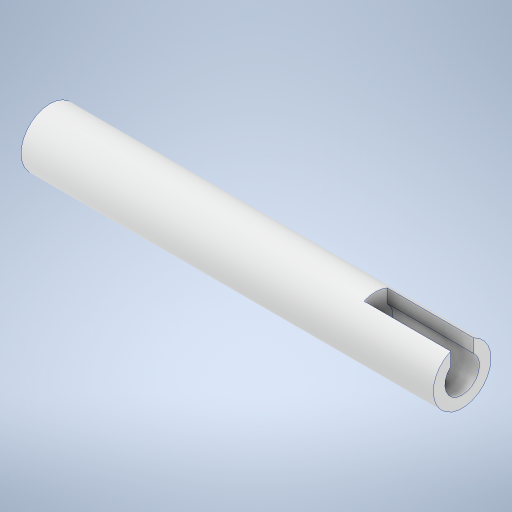
# Autodesk Inventor part: RZvector-arm-rotate-v1-Shaft-MM5-Shaft
Saved by Autodesk Inventor 2024 (Build 280153000, 153)
## iProperties
Created: 2024-03-13
Part Number: RZvector-arm-rotate-v1-Shaft-MM5-Shaft
Material: アルミニウム 6061
Document SubType Name: Modeling
Designer: haruy
Density: 2.7 g/cm^3
Appearance: アルミニウム - フラット
Author: haruy
Autodesk Inventor part; units mm, degrees
ref_plane "YZ Plane" through (0, 0, 0) normal (1, 0, 0) x (0, 1, 0)
ref_plane "XZ Plane" through (0, 0, 0) normal (0, 1, 0) x (-1, 0, 0)
ref_plane "XY Plane" through (0, 0, 0) normal (0, 0, 1) x (1, 0, 0)
sketch "スケッチ1" plane through (0, 0, 0) normal (1, 0, 0) x (0, 1, 0)
  circle A0 centre (0, 0) radius 5
  dimension "d0" = 10
  constraints: 1 centre point, 1 coincident
  measures "d0" diameter of A0
extrude "押し出し1" add sketch "スケッチ1" along normal blind 71.5
sketch "スケッチ2" plane through (71.5, 0, 0) normal (1, 0, 0) x (0, 0, -1)
  circle A0 centre (0, 0) radius 3
  line L0 (-2, 5.6235) -> (-2, 0.6448)
  line L1 (-2, 0.6448) -> (2, 0.6448)
  line L2 (2, 0.6448) -> (2, 6.3088)
  line L3 (-2, 5.6235) -> (2, 5.6235)
  point P0 (-2, 2.2361)
  point P1 (2, 2.2361)
  dimension "d3" = 6
  dimension "d4" = 2
  dimension "d5" = 2
  constraints: 8 end point, 3 perpendicular, 1 centre point, 1 coincident, 1 point on line, 1 vertical
  measures "d3" diameter of A0
  measures "d4" distance from line of L0 point (0, 0)
  measures "d5" distance from line of point (0, 0) L2
extrude "押し出し2" cut sketch "スケッチ2" against normal blind 15
